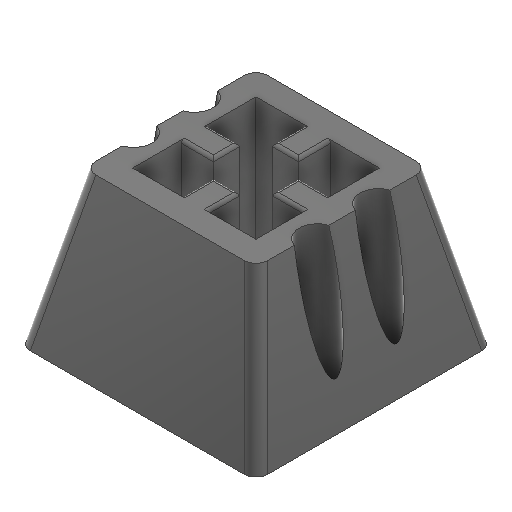
# Autodesk Inventor part: soporte base puente
Saved by Autodesk Inventor 2026.2 (Build 302298000, 298)
## iProperties
Created: 2026-04-27
Part Number: soporte base puente
Material: Genérico
Document SubType Name: Modeling
Designer: marti
Density: 1 g/cm^3
Appearance: Valor por defecto
Author: marti
Autodesk Inventor part; units mm, degrees
ref_plane "YZ Plane" through (0, 0, 0) normal (1, 0, 0) x (0, 1, 0)
ref_plane "XZ Plane" through (0, 0, 0) normal (0, 1, 0) x (-1, 0, 0)
ref_plane "XY Plane" through (0, 0, 0) normal (0, 0, 1) x (1, 0, 0)
sketch "Boceto1" plane through (0, 0, 0) normal (0, 1, 0) x (-1, 0, 0)
  line L0 (0, -38.9812) -> (38.9812, -38.9812)
  line L1 (38.9812, -38.9812) -> (-38.9812, -38.9812)
  line L2 (-38.9812, -38.9812) -> (-38.9812, 38.9812)
  line L3 (-38.9812, 38.9812) -> (38.9812, 38.9812)
  line L4 (38.9812, 38.9812) -> (38.9812, -38.9812)
  line L5 (0, -20.25) -> (20.25, -20.25)
  line L6 (20.25, -20.25) -> (-20.25, -20.25)
  line L7 (-20.25, -20.25) -> (-20.25, 20.25)
  line L8 (-20.25, 20.25) -> (20.25, 20.25)
  line L9 (20.25, 20.25) -> (20.25, -20.25)
  line L10 (-20.25, 4.3031) -> (-20.25, -4.3031)
  line L11 (0, 20.25) -> (4.3031, 20.25)
  line L12 (4.3031, 20.25) -> (-4.3031, 20.25)
  line L13 (4.3031, -20.25) -> (-4.3031, -20.25)
  line L14 (0, -20.25) -> (-4.225, -20.25)
  line L15 (-4.225, -20.25) -> (4.225, -20.25)
  line L16 (4.225, -20.25) -> (4.225, -9.75)
  line L17 (4.225, -9.75) -> (-4.225, -9.75)
  line L18 (-4.225, -9.75) -> (-4.225, -20.25)
  line L19 (4.225, 20.25) -> (4.225, 9.75)
  line L20 (4.225, 9.75) -> (-4.225, 9.75)
  line L21 (-4.225, 9.75) -> (-4.225, 20.25)
  line L22 (20.25, 0) -> (20.25, -4.225)
  line L23 (20.25, -4.225) -> (9.75, -4.225)
  line L24 (9.75, -4.225) -> (9.75, 4.225)
  line L25 (9.75, 4.225) -> (20.25, 4.225)
  line L26 (20.25, 4.225) -> (20.25, -4.225)
  line L27 (-20.25, -4.225) -> (-9.75, -4.225)
  line L28 (-9.75, -4.225) -> (-9.75, 4.225)
  line L29 (-9.75, 4.225) -> (-20.25, 4.225)
  line L30 (0, 0) -> (-30.15, 0)
  line L31 (-30.15, 0) -> (30.15, 0)
  line L32 (-30.15, 0) -> (-30.15, -10)
  circle A0 centre (-30.15, -10) radius 2.5
  circle A1 centre (-30.15, -10) radius 6
  line L33 (0, -7.25) -> (0, 4.225)
  circle A2 centre (-30.15, 10) radius 2.5
  circle A3 centre (-30.15, 10) radius 6
  circle A4 centre (30.15, -10) radius 2.5
  circle A5 centre (30.15, -10) radius 6
  circle A6 centre (30.15, 10) radius 6
  circle A7 centre (30.15, 10) radius 2.5
  circle A8 centre (30.15, -10) radius 2.5
  circle A9 centre (30.15, -10) radius 6
  circle A10 centre (30.15, 10) radius 2.5
  circle A11 centre (30.15, 10) radius 6
  circle A12 centre (-30.15, 10) radius 2.5
  circle A13 centre (-30.15, 10) radius 6
  circle A14 centre (-30.15, -10) radius 2.5
  circle A15 centre (-30.15, -10) radius 6
  dimension "d21" = 40.5
  dimension "d22" = 40.5
  dimension "d33" = 4.225
  dimension "d35" = 4.225
  dimension "d48" = 30.15
  dimension "d49" = 60.3
  dimension "d50" = 5
  dimension "d51" = 12
  dimension "d52" = 20
  dimension "d53" = 10
  constraints: 68 end point, 16 centre point, 13 coincident, 8 concentric, 8 parallel, 6 horizontal, 6 symmetric about line, 4 perpendicular, 4 point on line, 2 vertical, 1 midpoint, 6 other
  measures "d21" distance of L5.end L6.end
  measures "d22" distance of L6.end L7.end
  measures "d33" distance of L5.start L14.end
  measures "d35" distance of L22.start L22.end
  measures "d48" distance of L30.start L30.end
  measures "d49" distance of L30.end L31.end
  measures "d50" diameter of A0
  measures "d51" diameter of A1
  measures "d52" distance of A3.centre L32.end
  measures "d53" distance of L32.end L30.end
ref_plane "Plano de trabajo5" through (0, 50, 0) normal (0, 1, 0) x (1, 0, 0)
sketch "Boceto2" plane through (0, 50, 0) normal (0, 1, 0) x (1, 0, 0)
  point P0 (0, 0)
ref_plane "Plano de trabajo1" through (0, 0, 0) normal (0, -1, 0) x (1, 0, 0)
sketch "Boceto3" plane through (0, 0, 0) normal (0, -1, 0) x (1, 0, 0)
  point P0 (0, 0)
extrude "Extrusión4" add sketch "Boceto1" along normal blind 50 contours L1 L2 L3 L4 L0 | L6 L18 L17 L16 L5 | L23 L24 L31 L9 | L31 L24 L25 L9 | L7 L30 L28 L27 | L7 L29 L28 L30 | L19 L20 L21 L8
chamfer "Chaflán5" distance 10.75 distance2 50 5 edges at (0, 50, 38.9812) (38.9812, 50, 0) (-19.4906, 50, -38.9812) (19.4906, 50, -38.9812) (-38.9812, 50, 0) measured on face at (-19.4906, 50, -38.4812) measured on face at (19.4906, 50, -38.4812) measured on face at (38.4812, 50, 0) measured on face at (-38.4812, 50, 0) measured on face at (0, 50, 38.4812)
extrude "Extrusión5" add sketch "Boceto1" along normal blind 4.5 contours A1 | A3 | A5 | A6
fillet "Empalme4" radius 4 4 edges at (33.6063, 25, 33.6062) (33.6062, 25, -33.6063) (-33.6063, 25, -33.6062) (-33.6062, 25, 33.6063)
fillet "Empalme5" radius 1 24 edges at (15, 0, 4.225) (15, 0, -4.225) (9.75, 0, 0) (0, 0, 9.75) (4.225, 0, 15) (-4.225, 0, 15) (-15, 0, 4.225) (-9.75, 0, 0) (-15, 0, -4.225) (-4.225, 0, -15) (0, 0, -9.75) (4.225, 0, -15) (15, 50, 4.225) (15, 50, -4.225) (9.75, 50, 0) (0, 50, -9.75) (4.225, 50, -15) (-4.225, 50, -15) (-15, 50, -4.225) (-9.75, 50, 0) (-15, 50, 4.225) (-4.225, 50, 15) (4.225, 50, 15) (0, 50, 9.75)
